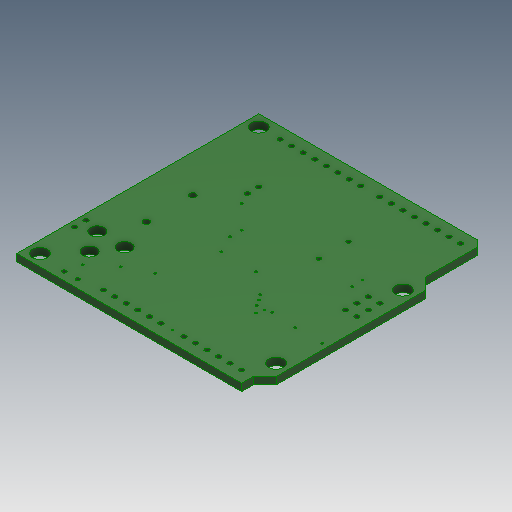
# Autodesk Inventor part: Arduino-Pro-v14.brd_Kontur
Saved by Autodesk Inventor 2017 (Build 210142000, 142)
## iProperties
Part Number: Arduino-Pro-v14.brd_Kontur
Material: Generisch
Document SubType Name: Modeling
Designer: Werkstatt
Density: 1 g/cm^3
Appearance: Board-Kontur
Author: Werkstatt
Autodesk Inventor part; units mm, degrees
ref_plane "YZ Plane" through (0, 0, 0) normal (1, 0, 0) x (0, 1, 0)
ref_plane "XZ Plane" through (0, 0, 0) normal (0, 1, 0) x (-1, 0, 0)
ref_plane "XY Plane" through (0, 0, 0) normal (0, 0, 1) x (1, 0, 0)
sketch "Skizze1" plane through (0, 0, 0) normal (0, 0, 1) x (1, 0, 0)
  line L0 (0, 53.34) -> (0, 0)
  line L1 (0, 0) -> (49.53, 0)
  line L2 (49.53, 0) -> (49.53, 2.54)
  line L3 (49.53, 2.54) -> (52.07, 5.08)
  line L4 (52.07, 5.08) -> (52.07, 38.1)
  line L5 (52.07, 38.1) -> (49.53, 40.64)
  line L6 (49.53, 40.64) -> (49.53, 52.07)
  line L7 (49.53, 52.07) -> (48.26, 53.34)
  line L8 (48.26, 53.34) -> (0, 53.34)
  circle A0 centre (34.29, 38.81) radius 0.45
  circle A1 centre (34.29, 32.31) radius 0.45
  circle A2 centre (46.99, 50.8) radius 0.51
  circle A3 centre (44.45, 50.8) radius 0.51
  circle A4 centre (41.91, 50.8) radius 0.51
  circle A5 centre (39.37, 50.8) radius 0.51
  circle A6 centre (36.83, 50.8) radius 0.51
  circle A7 centre (34.29, 50.8) radius 0.51
  circle A8 centre (31.75, 50.8) radius 0.51
  circle A9 centre (29.21, 50.8) radius 0.51
  circle A10 centre (34.29, 2.54) radius 0.51
  circle A11 centre (36.83, 2.54) radius 0.51
  circle A12 centre (39.37, 2.54) radius 0.51
  circle A13 centre (41.91, 2.54) radius 0.51
  circle A14 centre (44.45, 2.54) radius 0.51
  circle A15 centre (46.99, 2.54) radius 0.51
  circle A16 centre (25.02, 50.8) radius 0.51
  circle A17 centre (22.48, 50.8) radius 0.51
  circle A18 centre (19.94, 50.8) radius 0.51
  circle A19 centre (17.4, 50.8) radius 0.51
  circle A20 centre (14.86, 50.8) radius 0.51
  circle A21 centre (12.32, 50.8) radius 0.51
  circle A22 centre (9.78, 50.8) radius 0.51
  circle A23 centre (7.24, 50.8) radius 0.51
  circle A24 centre (16.51, 2.54) radius 0.51
  circle A25 centre (19.05, 2.54) radius 0.51
  circle A26 centre (21.59, 2.54) radius 0.51
  circle A27 centre (24.13, 2.54) radius 0.51
  circle A28 centre (26.67, 2.54) radius 0.51
  circle A29 centre (29.21, 2.54) radius 0.51
  circle A30 centre (46.99, 30.48) radius 0.51
  circle A31 centre (49.53, 30.48) radius 0.51
  circle A32 centre (46.99, 27.94) radius 0.51
  circle A33 centre (49.53, 27.94) radius 0.51
  circle A34 centre (46.99, 25.4) radius 0.51
  circle A35 centre (49.53, 25.4) radius 0.51
  circle A36 centre (4.65, 13.08) radius 1.5
  circle A37 centre (7.65, 8.38) radius 1.5
  circle A38 centre (10.65, 13.08) radius 1.5
  circle A39 centre (13.97, 36.83) radius 0.51
  circle A40 centre (13.97, 39.37) radius 0.51
  circle A41 centre (1.27, 11.43) radius 0.51
  circle A42 centre (1.27, 13.97) radius 0.51
  circle A43 centre (8.255, 30.48) radius 0.7
  circle A44 centre (8.255, 20.32) radius 0.7
  circle A45 centre (11.66, 1.778) radius 0.45
  circle A46 centre (8.66, 1.778) radius 0.45
  circle A47 centre (2.54, 50.8) radius 1.651
  circle A48 centre (2.54, 2.54) radius 1.651
  circle A49 centre (49.53, 35.56) radius 1.651
  circle A50 centre (49.53, 7.62) radius 1.651
  circle A51 centre (37.719, 14.986) radius 0.254
  circle A52 centre (29.845, 22.86) radius 0.254
  circle A53 centre (22.225, 22.86) radius 0.254
  circle A54 centre (44.831, 16.51) radius 0.254
  circle A55 centre (13.97, 8.89) radius 0.254
  circle A56 centre (35.56, 17.78) radius 0.254
  circle A57 centre (34.671, 18.923) radius 0.254
  circle A58 centre (9.398, 5.08) radius 0.254
  circle A59 centre (39.37, 16.891) radius 0.254
  circle A60 centre (31.75, 2.54) radius 0.254
  circle A61 centre (15.24, 34.29) radius 0.254
  circle A62 centre (20.32, 26.67) radius 0.254
  circle A63 centre (43.307, 30.607) radius 0.254
  circle A64 centre (36.322, 16.51) radius 0.254
  circle A65 centre (20.32, 29.21) radius 0.254
  circle A66 centre (43.18, 33.02) radius 0.254
  circle A67 centre (38.0746, 16.51) radius 0.254
  circle A68 centre (50.8, 16.51) radius 0.254
  circle A69 centre (19.05, 11.43) radius 0.254
  constraints: 70 centre point, 18 end point
extrude "Arduino-Pro-v14.brd_Kontur" add sketch "Skizze1" along normal blind 1.6
